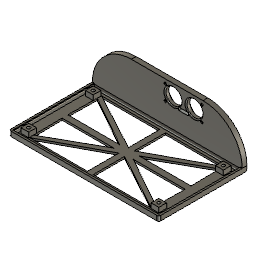
distance-sensor-enclosure (Autodesk Fusion 360 design; units mm, degrees)
Autodesk Fusion 360 part; units mm, degrees
sketch "pcb-base" plane through (0, 0, 0) normal (0, 0, 1) x (1, 0, 0)
  line L0 (-73.66, -40.64) -> (73.66, -40.64)
  line L1 (73.66, -40.64) -> (73.66, 40.64)
  line L2 (73.66, 40.64) -> (-73.66, 40.64)
  line L3 (-73.66, 40.64) -> (-73.66, -40.64)
  line L4 (-73.66, -40.64) -> (73.66, 40.64) construction
  line L5 (73.66, -40.64) -> (-73.66, 40.64) construction
  circle A0 centre (66.5764, 32.5141) radius 1.6
  line L6 (-73.66, 0) -> (73.66, 0) construction
  line L7 (0, 40.64) -> (0, -40.64) construction
  circle A1 centre (-66.5764, 32.5141) radius 1.6
  circle A2 centre (-66.5764, -32.5141) radius 1.6
  circle A3 centre (66.5764, -32.5141) radius 1.6
  dimension "d1" = 147.32
  dimension "d2" = 81.28
  dimension "d3" = 3.2
  dimension "d4" = 10.78
  constraint horizontal L0
  constraint perpendicular L0 L1
  constraint parallel L0 L2
  constraint parallel L1 L3
  constraint coincident L4 origin
  constraint coincident L5 origin
  constraint midpoint L3 L6.start
  constraint midpoint L1 L6.end
  constraint midpoint L2 L7.start
  constraint midpoint L0 L7.end
  constraint symmetric A0 L7 A1
  constraint symmetric A0 L6 A3
  constraint symmetric L6 A1 A2
  measures "d1" distance of L1.end L2.end
  measures "d2" distance of L0.end L1.end
  measures "d3" diameter of A0
  measures "d4" distance of L1.end A0.centre
sketch "box-frame" plane through (0, 0, 0) normal (0, 0, 1) x (1, 0, 0)
  line L0 (-76.66, -43.64) -> (76.66, -43.64)
  line L1 (76.66, -43.64) -> (76.66, 43.64)
  line L2 (76.66, 43.64) -> (-76.66, 43.64)
  line L3 (-76.66, 43.64) -> (-76.66, -43.64)
  line L4 (-76.66, -43.64) -> (76.66, 43.64) construction
  line L5 (76.66, -43.64) -> (-76.66, 43.64) construction
  dimension "d5" = 153.32
  dimension "d6" = 87.28
  constraint horizontal L0
  constraint perpendicular L0 L1
  constraint parallel L0 L2
  constraint parallel L1 L3
  constraint coincident L4 origin
  constraint coincident L5 origin
  measures "d5" distance of L1.end L2.end
  measures "d6" distance of L0.end L1.end
extrude "Extrude1" add sketch "box-frame" along normal blind 5 makes body 1
shell "Shell1" thickness 2 removed faces 1 at (25.5533, -14.5467, 5) on bodies 1
sketch "box-mounts" plane through (0, 0, 2) normal (0, 0, 1) x (-1, 0, 0)
  line L0 (74.66, -41.64) -> (74.66, 41.64)
  line L1 (74.66, 41.64) -> (-74.66, 41.64)
  line L2 (-74.66, 41.64) -> (-74.66, -41.64)
  line L3 (-74.66, -41.64) -> (74.66, -41.64)
  circle A0 centre (66.5764, -32.5141) radius 1.6
  circle A1 centre (-66.5764, -32.5141) radius 1.6
  circle A2 centre (-66.5764, 32.5141) radius 1.6
  circle A3 centre (66.5764, 32.5141) radius 1.6
  line L4 (70.5764, -28.5141) -> (62.5764, -28.5141)
  line L5 (62.5764, -28.5141) -> (62.5764, -36.5141)
  line L6 (62.5764, -36.5141) -> (70.5764, -36.5141)
  line L7 (70.5764, -36.5141) -> (70.5764, -28.5141)
  line L8 (70.5764, -28.5141) -> (62.5764, -36.5141) construction
  line L9 (62.5764, -28.5141) -> (70.5764, -36.5141) construction
  line L10 (0, -41.64) -> (0, 41.64) construction
  line L11 (74.66, 0) -> (-74.66, 0) construction
  line L12 (-74.66, 0) -> (74.66, 0) construction
  line L13 (-62.5764, -28.5141) -> (-62.5764, -36.5141)
  line L14 (-62.5764, -36.5141) -> (-70.5764, -36.5141)
  line L15 (-70.5764, -36.5141) -> (-70.5764, -28.5141)
  line L16 (-70.5764, -28.5141) -> (-62.5764, -28.5141)
  line L17 (62.5764, 28.5141) -> (62.5764, 36.5141)
  line L18 (70.5764, 28.5141) -> (62.5764, 28.5141)
  line L19 (70.5764, 36.5141) -> (70.5764, 28.5141)
  line L20 (62.5764, 36.5141) -> (70.5764, 36.5141)
  line L21 (-62.5764, 36.5141) -> (-70.5764, 36.5141)
  line L22 (-70.5764, 36.5141) -> (-70.5764, 28.5141)
  line L23 (-70.5764, 28.5141) -> (-62.5764, 28.5141)
  line L24 (-62.5764, 28.5141) -> (-62.5764, 36.5141)
  point P0 (-66.5764, 32.5141)
  point P1 (-66.5764, -32.5141)
  point P2 (66.5764, -32.5141)
  point P3 (66.5764, 32.5141)
  point P4 (66.5764, -32.5141)
  dimension "d10" = 8
  dimension "d11" = 8
  constraint horizontal L4
  constraint perpendicular L4 L5
  constraint parallel L4 L6
  constraint parallel L5 L7
  constraint coincident L8 P4
  constraint coincident L9 P4
  constraint coincident P4 P2
  constraint midpoint L3 L10.start
  constraint midpoint L1 L10.end
  constraint midpoint L0 L11.start
  constraint midpoint L2 L11.end
  constraint symmetric L4.start L10 L15.end
  constraint symmetric L4.end L10 L13.start
  constraint symmetric L5.end L10 L13.end
  constraint symmetric L6.end L10 L14.end
  constraint symmetric L10 L11.start L11.end
  constraint symmetric L10 L11.end L11.start
  constraint symmetric L4.start L11 L18.start
  constraint symmetric L4.end L11 L17.start
  constraint symmetric L5.end L11 L17.end
  constraint symmetric L6.end L11 L19.start
  constraint symmetric L11 L13.start L23.end
  constraint symmetric L11 L13.end L21.start
  constraint symmetric L11 L14.end L21.end
  constraint symmetric L11 L15.end L22.end
  measures "d10" distance of L5.end L6.end
  measures "d11" distance of L4.end L5.end
extrude "Extrude2" add sketch "box-mounts" along normal blind 5 separate body contours L4 L5 L6 L7 | L13 L14 L15 L16 | L17 L18 L19 L20 | L21 L22 L23 L24 makes body 2 at (66.6162, 35.7126, 2) makes body 3 at (66.6162, -29.3156, 2) makes body 4 at (-66.5365, 35.7126, 2) makes body 5 at (-66.5365, -29.3156, 2)
sketch "front-wall" plane through (0, 0, 5) normal (0, 0, 1) x (-1, 0, 0)
  line L0 (74.66, -41.64) -> (-74.66, -41.64)
  line L1 (-74.66, -41.64) -> (-74.66, 41.64)
  line L2 (-74.66, 41.64) -> (74.66, 41.64)
  line L3 (74.66, 41.64) -> (74.66, -41.64)
  line L4 (76.66, -43.64) -> (76.66, 43.64)
  line L5 (76.66, 43.64) -> (-76.66, 43.64)
  line L6 (-76.66, 43.64) -> (-76.66, -43.64)
  line L7 (-76.66, -43.64) -> (76.66, -43.64)
  line L8 (-76.66, -41.64) -> (76.66, -41.64)
  line L9 (76.66, -41.64) -> (76.66, -43.64)
  line L10 (76.66, -43.64) -> (-76.66, -43.64)
  line L11 (-76.66, -43.64) -> (-76.66, -41.64)
  constraint horizontal L8
  constraint vertical L9
  constraint horizontal L10
  constraint vertical L11
  constraint coincident L4.start L7.end
  constraint coincident L6 L8.start
extrude "Extrude3" add sketch "front-wall" along normal blind 40 contours L0 L4 L6 L7 L8 L9 L10 L11 bodies 3 2 1 4 5
sketch "hcsro4-cutout" plane through (0, 41.64, 0) normal (0, -1, 0) x (1, 0, 0)
  line L0 (-76.66, 45) -> (-76.66, 5)
  line L1 (-76.66, 5) -> (-74.66, 5)
  line L2 (-74.66, 5) -> (-74.66, 2)
  line L3 (-74.66, 2) -> (74.66, 2)
  line L4 (74.66, 2) -> (74.66, 5)
  line L5 (74.66, 5) -> (76.66, 5)
  line L6 (76.66, 5) -> (76.66, 45)
  line L7 (76.66, 45) -> (-76.66, 45)
  line L8 (-3.34, 23.9) -> (36.66, 23.9)
  line L9 (36.66, 23.9) -> (36.66, 42)
  line L10 (36.66, 42) -> (-3.34, 42)
  line L11 (-3.34, 42) -> (-3.34, 23.9)
  line L12 (-3.34, 23.9) -> (36.66, 42) construction
  line L13 (36.66, 23.9) -> (-3.34, 42) construction
  line L14 (16.66, 42) -> (16.66, 11.8) construction
  circle A0 centre (5.88, 32.9) radius 8.25
  circle A1 centre (27.44, 32.9) radius 8.25
  line L15 (36.66, 32.95) -> (-3.34, 32.95) construction
  circle A2 centre (-1.99, 40.65) radius 0.8
  circle A3 centre (35.31, 40.65) radius 0.8
  circle A4 centre (-1.99, 25.25) radius 0.8
  circle A5 centre (35.31, 25.25) radius 0.8
  line L16 (11.66, 23.9) -> (21.66, 23.9)
  line L17 (21.66, 23.9) -> (21.66, 26.9)
  line L18 (21.66, 26.9) -> (11.66, 26.9)
  line L19 (11.66, 26.9) -> (11.66, 23.9)
  point P0 (16.66, 32.95)
  dimension "d18" = 60
  dimension "d19" = 40
  dimension "d20" = 18.1
  dimension "d21" = 16.5
  dimension "d22" = 9.1
  dimension "d23" = 9.22
  dimension "d26" = 1.6
  dimension "d27" = 1.35
  dimension "d28" = 1.35
  dimension "d31" = 10
  dimension "d32" = 3
  dimension "d40" = 3
  constraint horizontal L8
  constraint perpendicular L8 L9
  constraint parallel L8 L10
  constraint parallel L9 L11
  constraint coincident L12 P0
  constraint coincident L13 P0
  constraint midpoint L10 L14.start
  constraint perpendicular L10 L14
  constraint symmetric L14 A0 A1
  constraint midpoint L9 L15.start
  constraint midpoint L11 L15.end
  constraint symmetric L14 A2 A3
  constraint symmetric L15 A2 A4
  constraint symmetric L15 A3 A5
  constraint horizontal L16
  constraint vertical L17
  constraint horizontal L18
  constraint vertical L19
  constraint coincident L8 L16.start
  constraint midpoint L14 L18
  measures "d18" distance of L6 P0
  measures "d19" distance of L9 L11
  measures "d20" distance of L8 L10
  measures "d21" diameter of A0
  measures "d22" distance of L10 A0.centre
  measures "d23" distance of L11 A0.centre
  measures "d26" diameter of A2
  measures "d27" distance of L10 A2.centre
  measures "d28" distance of L11 A2.centre
  measures "d31" distance of L16.start L16.end
  measures "d32" distance of L16.start L18.end
  measures "d40" distance of L7 L10
extrude "Extrude4" cut sketch "hcsro4-cutout" against normal blind 4 contours A0 | A1 bodies 4 2 5 3 1
extrude "Extrude5" cut sketch "hcsro4-cutout" against normal blind 2 contours A2 | A3 | A4 | A5 bodies 4 3 1 2 5
extrude "Extrude6" cut sketch "hcsro4-cutout" against normal blind 2 draft -20 contours L8 L16 L17 L18 L19 bodies 1
move_face "OffsetFaces1" offset 2 1 faces at (-52.0367, 43.64, 23.4167) on bodies 1
sketch "union-jack-cutout" plane through (0, 0, 2) normal (0, 0, 1) x (-1, 0, 0)
  line L0 (74.66, -41.64) -> (74.66, 41.64)
  line L1 (74.66, 41.64) -> (-74.66, 41.64)
  line L2 (-74.66, 41.64) -> (-74.66, -41.64)
  line L3 (-74.66, -41.64) -> (74.66, -41.64)
  line L4 (74.66, 0) -> (-74.66, 0) construction
  line L5 (0, 41.64) -> (0, -41) construction
  line L6 (62.5764, -32.5141) -> (63, -3)
  line L7 (63, -3) -> (10, -3)
  line L8 (10, -3) -> (62.5764, -32.5141)
  line L9 (10, 3) -> (62.5764, 32.5141)
  line L10 (62.5764, 32.5141) -> (63, 3)
  line L11 (63, 3) -> (10, 3)
  line L12 (-10, -3) -> (-62.5764, -32.5141)
  line L13 (-63, -3) -> (-10, -3)
  line L14 (-62.5764, -32.5141) -> (-63, -3)
  line L15 (-63, 3) -> (-10, 3)
  line L16 (-10, 3) -> (-62.5764, 32.5141)
  line L17 (-62.5764, 32.5141) -> (-63, 3)
  line L18 (3, -5) -> (3, -37)
  line L19 (3, -37) -> (62.5764, -37)
  line L20 (62.5764, -37) -> (3, -5)
  line L21 (-3, -37) -> (-62.5764, -37)
  line L22 (-3, -5) -> (-3, -37)
  line L23 (-62.5764, -37) -> (-3, -5)
  line L24 (3, 37) -> (62.5764, 37)
  line L25 (62.5764, 37) -> (3, 5)
  line L26 (3, 5) -> (3, 37)
  line L27 (-3, 5) -> (-3, 37)
  line L28 (-3, 37) -> (-62.5764, 37)
  line L29 (-62.5764, 37) -> (-3, 5)
  constraint midpoint L0 L4.start
  constraint midpoint L2 L4.end
  constraint midpoint L1 L5.start
  constraint perpendicular L1 L5
  constraint symmetric L4 L6.start L9.end
  constraint symmetric L4 L6.end L10.end
  constraint symmetric L4 L7.end L9.start
  constraint symmetric L5 L6.start L12.end
  constraint symmetric L5 L6.end L13.start
  constraint symmetric L5 L7.end L12.start
  constraint symmetric L5 L9.start L15.end
  constraint symmetric L5 L9.end L16.end
  constraint symmetric L5 L10.end L15.start
  constraint vertical L18
  constraint symmetric L5 L18.start L22.start
  constraint symmetric L5 L18.end L21.start
  constraint symmetric L5 L19.end L21.end
  constraint symmetric L4 L18.start L25.end
  constraint symmetric L4 L18.end L24.start
  constraint symmetric L4 L19.end L24.end
  constraint symmetric L4 L21.start L27.end
  constraint symmetric L4 L21.end L28.end
  constraint symmetric L4 L22.start L27.start
extrude "Extrude7" cut sketch "union-jack-cutout" against normal blind 2 contours L6 L7 L8 | L9 L10 L11 | L12 L13 L14 | L15 L16 L17 | L18 L19 L20 | L21 L22 L23 | L24 L25 L26 | L27 L28 L29 bodies 1 5 4 2 3
fillet "Fillet2" radius 40 2 edges at (-76.66, 43.64, 45) (76.66, 43.64, 45) on bodies 1
fillet "Fillet3" radius 2 2 edges at (76.66, -43.64, 2.5) (-76.66, -43.64, 2.5) on bodies 1
fillet "Fillet4" radius 2 1 edges at (0, 45.64, 0) on bodies 1
fillet "Fillet5" radius 2 1 edges at (0, 41.64, 2) on bodies 1
fillet "Fillet5" radius 2 3 edges at (-74.66, 0, 2) (0, -41.64, 2) (74.66, 0, 2) on bodies 1
fillet "Fillet6" radius 1 4 edges at (-1.8117, 41.64, 35.8833) (-1.8117, 45.64, 29.9167) (19.7483, 41.64, 35.8833) (19.7483, 45.64, 29.9167) on bodies 1
move_face "MoveFace1" to x (1, 0, 0) y (0, 1, 0) z (0, 0, 1) at (0, -1, 0) 12 faces at (66.6162, -29.3156, 7) (65.2431, -36.5141, 3.6667) (66.6163, -34.1136, 5.3333) (62.5764, -31.1807, 3.6667) (-65.2431, -36.5141, 3.6667) (-66.5365, -29.3156, 7) (-66.5365, -34.1136, 5.3333) (-70.5764, -33.8474, 3.6667) (70.5764, -33.8474, 3.6667) (-62.5764, -31.1807, 3.6667) (67.9097, -28.5141, 3.6667) (-67.9097, -28.5141, 3.6667) on bodies 3 5
fillet "Fillet7" radius 0.5 4 edges at (-2.7359, 41.64, 40.9393) (34.5641, 41.64, 40.9393) (34.5641, 41.64, 25.5393) (-2.7359, 41.64, 25.5393) on bodies 1
move_face "OffsetFaces2" offset 1 1 faces at (8.9162, 45.64, 9.2253) on bodies 1
equation "d5 = d1 + 6 mm"
equation "d6 = d2 + 6 mm"
